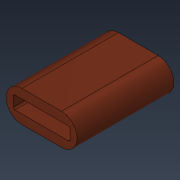
# Autodesk Inventor part: Kupferspule
Saved by Autodesk Inventor 2022.1 (Build 261234020, 234B)
## iProperties
Part Number: Kupferspule
Material: Kupfer
Document SubType Name: Modeling
Designer: rYan
Mass: 121.537 g
Surface Area: 75.5773 cm^2
Volume: 13.5948 cm^3
Density: 8.94 g/cm^3
Appearance: Kupfer - satiniert
Author: rYan
Autodesk Inventor part; units mm, degrees
ref_plane "YZ Plane" through (0, 0, 0) normal (1, 0, 0) x (0, 1, 0)
ref_plane "XZ Plane" through (0, 0, 0) normal (0, 1, 0) x (-1, 0, 0)
ref_plane "XY Plane" through (0, 0, 0) normal (0, 0, 1) x (1, 0, 0)
sketch "Skizze1" plane through (0, 0, 0) normal (0, 1, 0) x (-1, 0, 0)
  line L0 (12.8, 3.1) -> (-12.8, 3.1)
  line L1 (-13.6, 2.3) -> (-13.6, -2.3)
  line L2 (-12.8, -3.1) -> (12.8, -3.1)
  line L3 (13.6, -2.3) -> (13.6, 2.3)
  line L4 (13.6, 3.1) -> (-13.6, -3.1) construction
  line L5 (-13.6, 3.1) -> (13.6, -3.1) construction
  arc A0 (13.6, 2.3) -> (12.8, 3.1) centre (12.8, 2.3) ccw
  arc A1 (12.8, -3.1) -> (13.6, -2.3) centre (12.8, -2.3) ccw
  arc A2 (-13.6, -2.3) -> (-12.8, -3.1) centre (-12.8, -2.3) ccw
  arc A3 (-12.8, 3.1) -> (-13.6, 2.3) centre (-12.8, 2.3) ccw
  line L6 (9.5, 0) -> (-9.5, 0) construction
  line L7 (9.5, -7.5) -> (-9.5, -7.5)
  line L8 (-9.5, 7.5) -> (9.5, 7.5)
  arc A4 (9.5, -7.5) -> (9.5, 7.5) centre (9.5, 0) ccw
  arc A5 (-9.5, 7.5) -> (-9.5, -7.5) centre (-9.5, 0) ccw
  point P0 (0, 0)
  dimension "d0" = 27.2
  dimension "d1" = 6.2
  dimension "d2" = 0.8
  dimension "d6" = 4.4
  dimension "d7" = 34
  constraints: 20 end point, 12 point on circle, 12 tangent, 8 point on line, 6 centre point, 3 equal radius, 3 midpoint, 3 parallel, 2 horizontal, 1 perpendicular
  measures "d0" distance of L5.end L4.end
  measures "d1" distance of L4.end L5.start
  measures "d2" radius of A0
  measures "d6" distance between parallel lines of L8 L0
extrude "Extrusion1" add sketch "Skizze1" along normal mid plane 46.3
